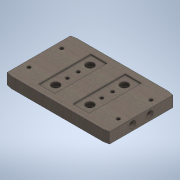
# Autodesk Inventor part: guidingplate
Saved by Autodesk Inventor 2022 (Build 260153000, 153)
## iProperties
Created: 2021-10-05
Part Number: guidingplate
Material: Generisch
Document SubType Name: Modeling
Designer: 123St
Density: 1 g/cm^3
Appearance: Walnuss
Author: 123St
Autodesk Inventor part; units mm, degrees
ref_plane "YZ Plane" through (0, 0, 0) normal (1, 0, 0) x (0, 1, 0)
ref_plane "XZ Plane" through (0, 0, 0) normal (0, 1, 0) x (-1, 0, 0)
ref_plane "XY Plane" through (0, 0, 0) normal (0, 0, 1) x (1, 0, 0)
sketch "Skizze1" plane through (0, 0, 0) normal (0, 1, 0) x (-1, 0, 0)
  line L0 (77.2474, 30) -> (-16.7526, 30)
  line L1 (-16.7526, 30) -> (-16.7526, -30)
  line L2 (-16.7526, -30) -> (77.2474, -30)
  line L3 (77.2474, -30) -> (77.2474, 30)
  line L4 (-35.5526, 0) -> (96.0474, 0) projected
  point P0 (0, 0)
  dimension "d0" = 30
  dimension "d1" = 60
  dimension "d2" = 94
  constraints: 8 end point, 2 parallel, 1 horizontal, 1 perpendicular
  measures "d0" distance between parallel lines of L2 L4
  measures "d1" distance between parallel lines of L2 L0
  measures "d2" distance between parallel lines of L1 L3
extrude "Extrusion1" add sketch "Skizze1" along normal blind 10
sketch "Skizze4" plane through (0, 10, 0) normal (0, 1, 0) x (1, 0, 0)
  circle A0 centre (-14.4974, -15.75) radius 2
  circle A1 centre (-14.4974, 15.75) radius 2
  circle A2 centre (-45.9974, -15.75) radius 2
  circle A3 centre (-45.9974, 15.75) radius 2
  line L0 (35.5526, 0) -> (-96.0474, 0) projected
  line L1 (16.7526, -30) -> (16.7526, 30) projected
  line L2 (-77.2474, 30) -> (-77.2474, -30) projected
  point P0 (0, 0)
  dimension "d21" = 4
  dimension "d22" = 15.75
  dimension "d23" = 15.75
  dimension "d26" = 15.75
  dimension "d27" = 15.75
  dimension "d30" = 4
  dimension "d31" = 4
  dimension "d32" = 4
  dimension "d127" = 31.5
  dimension "d128" = 31.5
  dimension "d129" = 31.25
  dimension "d130" = 31.25
  constraints: 4 centre point
  measures "d21" diameter of A0
  measures "d22" distance from line of L0 A0.centre
  measures "d23" distance from line of L0 A1.centre
  measures "d26" distance from line of L0 A2.centre
  measures "d27" distance from line of L0 A3.centre
  measures "d30" diameter of A1
  measures "d31" diameter of A2
  measures "d32" diameter of A3
  measures "d127" distance of A1.centre A3.centre
  measures "d128" distance of A2.centre A0.centre
  measures "d129" distance from line of A2.centre L2
  measures "d130" distance from line of L2 A3.centre
extrude "Extrusion4" cut sketch "Skizze4" against normal blind 10
sketch "Skizze5" plane through (0, 10, 0) normal (0, 1, 0) x (1, 0, 0)
  line L0 (-6.9974, -24) -> (-21.9974, -24)
  line L1 (-21.9974, -24) -> (-21.9974, 24)
  line L2 (-21.9974, 24) -> (-6.9974, 24)
  line L3 (-6.9974, 24) -> (-6.9974, -24)
  line L4 (-38.4974, 24) -> (-53.4974, 24)
  line L5 (-53.4974, 24) -> (-53.4974, -24)
  line L6 (-53.4974, -24) -> (-38.4974, -24)
  line L7 (-38.4974, -24) -> (-38.4974, 24)
  line L8 (35.5526, 0) -> (-96.0474, 0) projected
  line L9 (16.7526, -30) -> (16.7526, 30) projected
  line L10 (-77.2474, 30) -> (-77.2474, -30) projected
  point P0 (0, 0)
  dimension "d35" = 15
  dimension "d36" = 48
  dimension "d37" = 24
  dimension "d38" = 23.75
  dimension "d39" = 15
  dimension "d40" = 23.75
  constraints: 16 end point, 4 parallel, 2 horizontal, 2 perpendicular, 2 point on line
  measures "d35" distance between parallel lines of L3 L1
  measures "d36" distance between parallel lines of L2 L0
  measures "d37" distance between parallel lines of L8 L2
  measures "d38" distance between parallel lines of L9 L3
  measures "d39" distance of L5.end L6.end
  measures "d40" distance between parallel lines of L10 L5
extrude "Extrusion5" cut sketch "Skizze5" against normal blind 1
sketch "Skizze6" plane through (0, 9, 0) normal (0, 1, 0) x (1, 0, 0)
  circle A0 centre (-14.4974, -15.75) radius 3.6
  circle A1 centre (-14.4974, 15.75) radius 3.6
  circle A2 centre (-45.9974, -15.75) radius 3.6
  circle A3 centre (-45.9974, 15.75) radius 3.6
  circle A4 centre (-45.9974, 15.75) radius 2 projected
  circle A5 centre (-45.9974, -15.75) radius 2 projected
  circle A6 centre (-14.4974, 15.75) radius 2 projected
  circle A7 centre (-14.4974, -15.75) radius 2 projected
  circle A8 centre (-3.2474, -15.75) radius 3.6
  circle A9 centre (-3.2474, 15.75) radius 3.6
  circle A10 centre (-45.9974, -15.75) radius 3.6
  circle A11 centre (-53.2474, 15.75) radius 3.6
  circle A12 centre (-53.2474, 15.75) radius 2
  circle A13 centre (-45.9974, -15.75) radius 2
  circle A14 centre (-3.2474, 15.75) radius 2
  circle A15 centre (-3.2474, -15.75) radius 2
  circle A16 centre (-3.2474, -15.75) radius 3.6
  circle A17 centre (-3.2474, 15.75) radius 3.6
  circle A18 centre (-45.9974, -15.75) radius 3.6
  circle A19 centre (-53.2474, 15.75) radius 3.6
  circle A20 centre (-53.2474, 15.75) radius 2
  circle A21 centre (-45.9974, -15.75) radius 2
  circle A22 centre (-3.2474, 15.75) radius 2
  circle A23 centre (-3.2474, -15.75) radius 2
  circle A24 centre (-3.2474, -15.75) radius 3.6
  circle A25 centre (-3.2474, 15.75) radius 3.6
  circle A26 centre (-53.2474, -15.75) radius 3.6
  circle A27 centre (-53.2474, 15.75) radius 3.6
  circle A28 centre (-53.2474, 15.75) radius 2
  circle A29 centre (-53.2474, -15.75) radius 2
  circle A30 centre (-3.2474, 15.75) radius 2
  circle A31 centre (-3.2474, -15.75) radius 2
  line L0 (-77.2474, 30) -> (-77.2474, -30) projected
  point P0 (0, 0)
  point P1 (0, 0)
  point P2 (0, 0)
  point P3 (0, 0)
  point P4 (-45.7474, 16.7182)
  point P5 (-45.7474, 14.7818)
  point P6 (-45.7474, -14.7818)
  point P7 (-45.7474, -16.7182)
  point P8 (-10.7474, 14.7818)
  point P9 (-10.7474, 16.7182)
  point P10 (-10.7474, -16.7182)
  point P11 (-10.7474, -14.7818)
  dimension "d43" = 7.2
  dimension "d44" = 7.2
  dimension "d45" = 7.2
  dimension "d46" = 7.2
  dimension "d79" = 7.2
  dimension "d80" = 7.2
  dimension "d81" = 7.2
  dimension "d82" = 7.2
  dimension "d83" = 7.2
  dimension "d84" = 7.2
  dimension "d85" = 7.2
  dimension "d86" = 7.2
  dimension "d87" = 7.2
  dimension "d88" = 7.2
  dimension "d89" = 7.2
  dimension "d90" = 7.2
  dimension "d142" = 31.25
  dimension "d143" = 31.25
  constraints: 28 centre point, 12 concentric, 8 other
  measures "d43" diameter of A0
  measures "d44" diameter of A1
  measures "d45" diameter of A2
  measures "d46" diameter of A3
  measures "d79" diameter of A8
  measures "d80" diameter of A9
  measures "d81" diameter of A10
  measures "d82" diameter of A11
  measures "d83" diameter of A16
  measures "d84" diameter of A17
  measures "d85" diameter of A18
  measures "d86" diameter of A19
  measures "d87" diameter of A24
  measures "d88" diameter of A25
  measures "d89" diameter of A26
  measures "d90" diameter of A27
  measures "d142" distance from line of L0 A10.centre
  measures "d143" distance from line of L0 A18.centre
extrude "Extrusion6" cut sketch "Skizze6" against normal blind 3 contours A0 | A1 | A2 | A3 | A4 | A5 | A6 | A7
sketch "Skizze8" plane through (0, 9, 0) normal (0, 1, 0) x (1, 0, 0)
  circle A0 centre (-14.4974, -5.0565) radius 1.5
  circle A1 centre (-14.4974, 4.9435) radius 1.5
  circle A2 centre (-45.9974, -5.0565) radius 1.5
  circle A3 centre (-45.9974, 4.9435) radius 1.5
  line L0 (-77.2474, 30) -> (-77.2474, -30) projected
  line L1 (16.7526, -30) -> (16.7526, 30) projected
  point P0 (0, 0)
  dimension "d56" = 10
  dimension "d57" = 10
  dimension "d58" = 31.25
  dimension "d59" = 31.25
  dimension "d62" = 3
  dimension "d63" = 3
  dimension "d64" = 3
  dimension "d65" = 3
  dimension "d146" = 31.25
  constraints: 4 centre point
  measures "d56" distance of A1.centre A0.centre
  measures "d57" distance of A3.centre A2.centre
  measures "d58" distance from line of L0 A2.centre
  measures "d59" distance from line of L0 A3.centre
  measures "d62" diameter of A0
  measures "d63" diameter of A1
  measures "d64" diameter of A2
  measures "d65" diameter of A3
  measures "d146" distance from line of L1 A1.centre
extrude "Extrusion7" cut sketch "Skizze8" against normal blind 10
chamfer "Fase1" distance 0.5 angle 45 4 edges at (-47.9974, 6, 15.75) (-47.9974, 6, -15.75) (-16.4974, 6, -15.75) (-16.4974, 6, 15.75)
sketch "Skizze9" plane through (0, 0, 0) normal (0, -1, 0) x (1, 0, 0)
  line L0 (-6.9974, -24) -> (-21.9974, -24)
  line L1 (-21.9974, -24) -> (-21.9974, 24)
  line L2 (-21.9974, 24) -> (-6.9974, 24)
  line L3 (-6.9974, 24) -> (-6.9974, -24)
  line L4 (-38.4974, 24) -> (-53.4974, 24)
  line L5 (-53.4974, 24) -> (-53.4974, -24)
  line L6 (-53.4974, -24) -> (-38.4974, -24)
  line L7 (-38.4974, -24) -> (-38.4974, 24)
  line L8 (34.7526, 0) -> (-91.2474, 0)
  line L9 (16.7526, 30) -> (16.7526, -30) projected
  line L10 (-77.2474, -30) -> (-77.2474, 30) projected
  point P0 (0, 0)
  point P1 (0, 0)
  dimension "d71" = 15
  dimension "d72" = 48
  dimension "d73" = 24
  dimension "d75" = 15
  dimension "d144" = 23.75
  dimension "d145" = 23.75
  constraints: 18 end point, 4 parallel, 2 horizontal, 2 perpendicular, 2 point on line
  measures "d71" distance between parallel lines of L3 L1
  measures "d72" distance between parallel lines of L2 L0
  measures "d73" distance between parallel lines of L8 L2
  measures "d75" distance of L5.end L6.end
  measures "d144" distance between parallel lines of L9 L3
  measures "d145" distance between parallel lines of L10 L5
extrude "Extrusion8" cut sketch "Skizze9" against normal blind 1
sketch "Skizze10" plane through (0, 0, 0) normal (0, -1, 0) x (1, 0, 0)
  circle A0 centre (-14.4974, -15.75) radius 3.6
  circle A1 centre (-14.4974, 15.75) radius 3.6
  circle A2 centre (-45.9974, -15.75) radius 3.6
  circle A3 centre (-45.9974, 15.75) radius 3.6
  circle A4 centre (-45.9974, 15.75) radius 2
  circle A5 centre (-45.9974, -15.75) radius 2
  circle A6 centre (-14.4974, 15.75) radius 2
  circle A7 centre (-14.4974, -15.75) radius 2
  circle A8 centre (-3.2474, -15.75) radius 3.6
  circle A9 centre (-3.2474, 15.75) radius 3.6
  circle A10 centre (-45.9974, -15.75) radius 3.6
  circle A11 centre (-53.2474, 15.75) radius 3.6
  circle A12 centre (-53.2474, 15.75) radius 2
  circle A13 centre (-45.9974, -15.75) radius 2
  circle A14 centre (-3.2474, 15.75) radius 2
  circle A15 centre (-3.2474, -15.75) radius 2
  circle A16 centre (-3.2474, -15.75) radius 3.6
  circle A17 centre (-3.2474, 15.75) radius 3.6
  circle A18 centre (-53.2474, -15.75) radius 3.6
  circle A19 centre (-53.2474, 15.75) radius 3.6
  circle A20 centre (-53.2474, 15.75) radius 2
  circle A21 centre (-53.2474, -15.75) radius 2
  circle A22 centre (-3.2474, 15.75) radius 2
  circle A23 centre (-3.2474, -15.75) radius 2
  circle A24 centre (-3.2474, -15.75) radius 3.6
  circle A25 centre (-3.2474, 15.75) radius 3.6
  circle A26 centre (-53.2474, -15.75) radius 3.6
  circle A27 centre (-53.2474, 15.75) radius 3.6
  circle A28 centre (-53.2474, 15.75) radius 2
  circle A29 centre (-53.2474, -15.75) radius 2
  circle A30 centre (-3.2474, 15.75) radius 2
  circle A31 centre (-3.2474, -15.75) radius 2
  line L0 (-77.2474, -30) -> (-77.2474, 30) projected
  line L1 (16.7526, 30) -> (16.7526, -30) projected
  point P0 (0, 0)
  point P1 (0, 0)
  point P2 (0, 0)
  point P3 (0, 0)
  point P4 (0, 0)
  dimension "d91" = 7.2
  dimension "d92" = 7.2
  dimension "d93" = 7.2
  dimension "d94" = 7.2
  dimension "d95" = 7.2
  dimension "d96" = 7.2
  dimension "d97" = 7.2
  dimension "d98" = 7.2
  dimension "d99" = 7.2
  dimension "d100" = 7.2
  dimension "d101" = 7.2
  dimension "d102" = 7.2
  dimension "d103" = 7.2
  dimension "d104" = 7.2
  dimension "d105" = 7.2
  dimension "d106" = 7.2
  dimension "d147" = 31.25
  dimension "d148" = 31.25
  dimension "d149" = 31.25
  dimension "d150" = 31.25
  dimension "d151" = 31.25
  constraints: 32 centre point, 16 concentric
  measures "d91" diameter of A0
  measures "d92" diameter of A1
  measures "d93" diameter of A2
  measures "d94" diameter of A3
  measures "d95" diameter of A8
  measures "d96" diameter of A9
  measures "d97" diameter of A10
  measures "d98" diameter of A11
  measures "d99" diameter of A16
  measures "d100" diameter of A17
  measures "d101" diameter of A18
  measures "d102" diameter of A19
  measures "d103" diameter of A24
  measures "d104" diameter of A25
  measures "d105" diameter of A26
  measures "d106" diameter of A27
  measures "d147" distance from line of L0 A3.centre
  measures "d148" distance from line of L0 A10.centre
  measures "d149" distance from line of L1 A1.centre
  measures "d150" distance from line of L1 A0.centre
  measures "d151" distance from line of L0 A2.centre
extrude "Extrusion9" cut sketch "Skizze10" against normal blind 4 contours A0 | A1 | A2 | A3 | A4 | A5 | A6 | A7
sketch "Skizze12" plane through (0, 10, 0) normal (0, 1, 0) x (1, 0, 0)
  circle A0 centre (-71.2474, -15) radius 1.5
  circle A1 centre (-71.2474, 15) radius 1.5
  circle A2 centre (10.7526, 15) radius 1.5
  circle A3 centre (10.7526, -15) radius 1.5
  line L0 (-77.2474, 30) -> (-77.2474, -30) projected
  line L1 (16.7526, -30) -> (16.7526, 30) projected
  point P0 (0, 0)
  dimension "d121" = 3
  dimension "d122" = 3
  dimension "d123" = 3
  dimension "d124" = 3
  dimension "d131" = 82
  dimension "d132" = 82
  dimension "d138" = 6
  dimension "d139" = 6
  constraints: 4 centre point
  measures "d121" diameter of A0
  measures "d122" diameter of A1
  measures "d123" diameter of A2
  measures "d124" diameter of A3
  measures "d131" distance of A2.centre A1.centre
  measures "d132" distance of A3.centre A0.centre
  measures "d138" distance from line of L0 A0.centre
  measures "d139" distance from line of L0 A1.centre
extrude "Extrusion11" cut sketch "Skizze12" against normal blind 60
sketch "Skizze15" plane through (-77.2474, 0, -30) normal (-1, 0, 0) x (0, 0, 1)
  circle A0 centre (38, 5) radius 1.15
  circle A1 centre (22, 5) radius 1.15
  line L0 (30, 12) -> (30, -2) projected
  line L1 (0, 10) -> (60, 10) projected
  point P0 (30, 0)
  dimension "d158" = 8
  dimension "d159" = 8
  dimension "d160" = 5
  dimension "d163" = 2.3
  dimension "d164" = 2.3
  constraints: 2 centre point
  measures "d158" distance from line of L0 A1.centre
  measures "d159" distance from line of L0 A0.centre
  measures "d160" distance from line of L1 A1.centre
  measures "d163" diameter of A1
  measures "d164" diameter of A0
extrude "Extrusion13" cut sketch "Skizze15" against normal blind 10
chamfer "Fase2" distance 2 angle 45 2 edges at (-77.2474, 5, 6.85) (-77.2474, 5, -9.15)
sketch "Skizze16" plane through (16.7526, 0, 30) normal (1, 0, 0) x (0, 0, -1)
  circle A0 centre (38, 5) radius 1.15
  circle A1 centre (22, 5) radius 1.15
  line L0 (0, 10) -> (60, 10) projected
  line L1 (30, -2) -> (30, 12) projected
  point P0 (30, 0)
  dimension "d168" = 5
  dimension "d169" = 5
  dimension "d170" = 8
  dimension "d171" = 8
  dimension "d172" = 2.3
  dimension "d173" = 2.3
  constraints: 2 centre point
  measures "d168" distance from line of A0.centre L0
  measures "d169" distance from line of L0 A1.centre
  measures "d170" distance from line of L1 A0.centre
  measures "d171" distance from line of L1 A1.centre
  measures "d172" diameter of A0
  measures "d173" diameter of A1
extrude "Extrusion14" cut sketch "Skizze16" against normal blind 10
chamfer "Fase3" distance 2 angle 45 2 edges at (16.7526, 5, 9.15) (16.7526, 5, -6.85)
sketch "Skizze17" plane through (0, 0, 0) normal (0, -1, 0) x (1, 0, 0)
  line L0 (16.7526, 30) -> (11.7526, 30)
  line L1 (16.7526, 29) -> (11.7526, 30)
  line L2 (16.7526, 29) -> (16.7526, 30)
  line L3 (16.7526, -30) -> (11.7526, -30)
  line L4 (16.7526, -29) -> (11.7526, -30)
  line L5 (16.7526, -29) -> (16.7526, -30)
  line L6 (-77.2474, -30) -> (-72.2474, -30)
  line L7 (-77.2474, -30) -> (-77.2474, -29)
  line L8 (-77.2474, -29) -> (-72.2474, -30)
  line L9 (-77.2474, 30) -> (-72.2474, 30)
  line L10 (-77.2474, 30) -> (-77.2474, 29)
  line L11 (-77.2474, 29) -> (-72.2474, 30)
  point P0 (0, 0)
  dimension "d179" = 1
  dimension "d180" = 5
  dimension "d181" = 5
  dimension "d182" = 1
  dimension "d183" = 1
  dimension "d184" = 5
  dimension "d185" = 5
  dimension "d186" = 1
  constraints: 24 end point, 2 perpendicular, 2 point on line
  measures "d179" distance of L9.start L10.end
  measures "d180" distance of L9.start L9.end
  measures "d181" distance of L0.start L0.end
  measures "d182" distance of L1.start L0.start
  measures "d183" distance of L4.start L3.start
  measures "d184" distance of L3.start L3.end
  measures "d185" distance of L6.start L6.end
  measures "d186" distance of L6.start L7.end
extrude "Extrusion15" cut sketch "Skizze17" against normal blind 10
